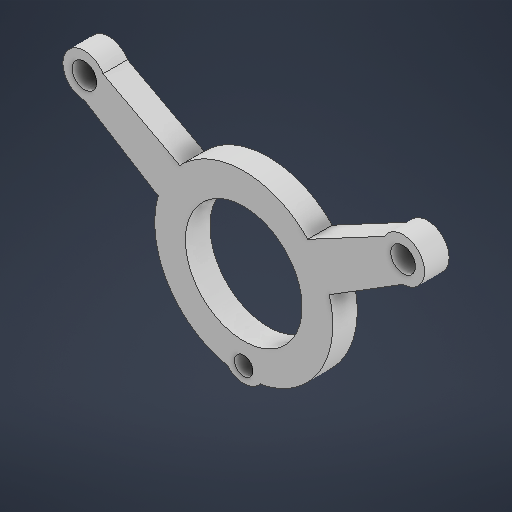
# Autodesk Inventor part: Tri
Saved by Autodesk Inventor 2025.3 (Build 293356000, 356)
## iProperties
Created: 2025-04-20
Part Number: Tri
Material: Generic
Document SubType Name: Modeling
Designer: Nelson
Density: 1 g/cm^3
Appearance: Default
Author: Nelson
Autodesk Inventor part; units mm, degrees
ref_plane "YZ Plane" through (0, 0, 0) normal (1, 0, 0) x (0, 1, 0)
ref_plane "XZ Plane" through (0, 0, 0) normal (0, 1, 0) x (-1, 0, 0)
ref_plane "XY Plane" through (0, 0, 0) normal (0, 0, 1) x (1, 0, 0)
sketch "Sketch1" plane through (0, 0, 0) normal (0, 0, 1) x (1, 0, 0)
  circle A0 centre (0, 0) radius 9.5
  circle A1 centre (0, 0) radius 14.5
  line L0 (0, 0) -> (25.9808, 15)
  line L1 (0, 0) -> (-25.9808, 15)
  line L2 (-21, 0) -> (21, 0) construction
  line L3 (0, 0) -> (0, -15.6153)
  circle A2 centre (-25.9808, 15) radius 3.5
  circle A3 centre (25.9808, 15) radius 3.5
  line L4 (-25.9808, 11.5) -> (-13.9374, 4)
  line L5 (-22.9497, 16.75) -> (-10.4328, 10.0701)
  line L6 (25.9808, 11.5) -> (13.9374, 4)
  line L7 (22.9497, 16.75) -> (10.4328, 10.0701)
  circle A4 centre (-25.9808, 15) radius 2
  circle A5 centre (25.9808, 15) radius 2
  line L8 (0, -16.5) -> (0, -13)
  circle A6 centre (0, -12) radius 2.5
  circle A7 centre (0, -12) radius 3.5
  line L9 (0, -12) -> (0, -13)
  circle A8 centre (0, -13) radius 1.5
  point P0 (-22.9497, 16.75)
  point P1 (25.9808, 11.5)
  point P2 (22.9497, 16.75)
  point P3 (2.1651, -9.25)
  point P4 (0, -9.5)
  point P5 (-2.681, -14.25)
  point P6 (2.681, -14.25)
  dimension "d1" = 29
  dimension "d8" = 7
  dimension "d0" = 19
  dimension "d2" = 30
  dimension "d3" = 30
  dimension "d6" = 120
  dimension "d7" = 120
  dimension "d9" = 7
  dimension "d12" = 4
  dimension "d13" = 4
  dimension "d15" = 3.5
  dimension "d17" = 5
  dimension "d18" = 7
  dimension "d19" = 1
  dimension "d20" = 3
  constraints: 20 end point, 8 coincident, 7 centre point, 6 symmetric about line, 2 point on line, 1 collinear, 1 horizontal, 1 midpoint, 1 vertical, 6 other
  measures "d0" diameter of A0
  measures "d2" distance of L0.start L0.end
  measures "d3" distance of L0.start L1.end
  measures "d6" angle of L0 L3
  measures "d7" angle of L1 L3
  measures "d9" diameter of A3
  measures "d12" diameter of A4
  measures "d13" diameter of A5
  measures "d15" distance of L8.start L8.end
  measures "d17" diameter of A6
  measures "d18" diameter of A7
  measures "d19" distance of L9.start L8.end
  measures "d20" diameter of A8
extrude "Extrusion1" add sketch "Sketch1" along normal blind 4 contours A0 L0 A1 A7 | A0 L1 A1 L0 | A7 A1 A6 A0 | A0 A7 A1 L1 | L0 A3 L6 A1 | A1 L7 A3 L0 | A6 A1 A7 A0 | A6 A8 L3 | L3 A8 A6 | L1 A2 L5 A1 | A1 L4 A2 L1 | A3 | L3 A7 A1 | A1 A7 L3 | A2
body "Solid1"
